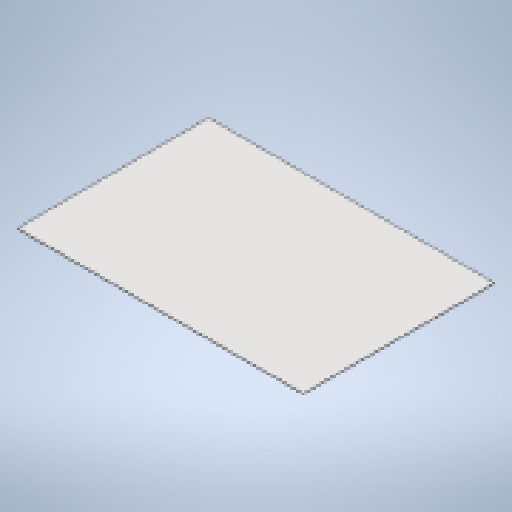
# Autodesk Inventor part: BSH 015 board cone 5
Saved by Autodesk Inventor 2025 (Build 290162010, 162A)
## iProperties
Created: 2024-07-23
Part Number: BSH 015 board cone 5
Material: 09g2s
Document SubType Name: Sheet Metal
Designer: admin
Mass: 40581.4 g
Surface Area: 34651.2 cm^2
Volume: 5169.6 cm^3
Density: 7.85 g/cm^3
Flat Pattern Width: 134.5 cm
Flat Pattern Length: 90 cm
Flat Pattern Area: 12105 cm^2
Sheet Metal Rule: AISI304 3mm Die 32
Sheet Metal Width: 1345,000 mm
Sheet Metal Length: 900,000 mm
Sheet Metal Area: 1210500,000 mm^2
Appearance: Default
Author: admin
Autodesk Inventor part; units mm, degrees
ref_plane "YZ Plane" through (0, 0, 0) normal (1, 0, 0) x (0, 1, 0)
ref_plane "XZ Plane" through (0, 0, 0) normal (0, 1, 0) x (-1, 0, 0)
ref_plane "XY Plane" through (0, 0, 0) normal (0, 0, 1) x (1, 0, 0)
sketch "Sketch1" plane through (0, 0, 0) normal (0, 0, 1) x (1, 0, 0)
  line L0 (0, -450) -> (1345, -450)
  line L1 (1345, -450) -> (1345, 450)
  line L2 (1345, 450) -> (0, 450)
  line L3 (0, 450) -> (0, -450)
  point P0 (0, 0)
  point P1 (0, 0)
  dimension "d0" = 1345
  dimension "d1" = 900
  measures "d0" distance of L2.end L1.end
  measures "d1" distance of L1.end L0.end
extrude "Plate1" add sketch "Sketch1" along normal blind 3
equation "\"d2\" = Thickness"
equation "\"BendReliefWidth\" = Thickness"
equation "\"BendReliefDepth\" = 0.5 * Thickness"
equation "\"CornerReliefSize\" = 4 * Thickness"
equation "\"MinimumRemnant\" = 2 * Thickness"
equation "\"TransitionRadius\" = BendRadius"
equation "\"JacobiRadiusSize\" = BendRadius"
equation "\"GapSize\" = Thickness"
equation "\"Thickness\" = 3"
equation "\"BendRadius\" = 5"
body "Solid1"
